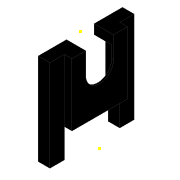
# Autodesk Inventor part: vertical_face_block
Saved by Autodesk Inventor 2019 (Build 230136000, 136)
## iProperties
Created: 2023-11-20
Part Number: vertical_face_block
Material: Aluminum 6061
Document SubType Name: Modeling
Designer: prich
Density: 2.7 g/cm^3
Appearance: Aluminum - Flat
Mass: 329.506 g
Surface Area: 342.022 cm^2
Volume: 122.039 cm^3
Author: prich
Autodesk Inventor part; units mm, degrees
ref_plane "YZ Plane" through (0, 0, 0) normal (1, 0, 0) x (0, 1, 0)
ref_plane "XZ Plane" through (0, 0, 0) normal (0, 1, 0) x (-1, 0, 0)
ref_plane "XY Plane" through (0, 0, 0) normal (0, 0, 1) x (1, 0, 0)
sketch "Sketch1" plane through (0, 0, 0) normal (0, 1, 0) x (-1, 0, 0)
  line L0 (0.0752, 55.5625) -> (-25.3248, 55.5625)
  line L1 (-25.3248, 55.5625) -> (-25.3248, -55.5625)
  line L2 (-25.3248, -55.5625) -> (0.0752, -55.5625)
  line L3 (0.0752, -55.5625) -> (0.0752, 55.5625)
  line L4 (54.9786, 0) -> (-47.41, 0) construction
  point P0 (0, 0)
  dimension "d0" = 111.125
  dimension "d1" = 25.4
  constraints: 10 end point, 2 horizontal, 2 parallel, 1 perpendicular, 1 other
  measures "d0" distance between parallel lines of L2 L0
  measures "d1" distance between parallel lines of L1 L3
extrude "Extrusion1" add sketch "Sketch1" along normal blind 120.65
sketch "Sketch2" plane through (25.3248, 0, 55.5625) normal (1, 0, 0) x (0, 0, -1)
  line L0 (55.5625, 0) -> (55.5625, 120.65) construction
  line L1 (0, 120.65) -> (111.125, 120.65) construction
  line L2 (19.05, 120.65) -> (92.075, 120.65)
  line L3 (92.075, 120.65) -> (92.075, 38.1)
  line L4 (92.075, 38.1) -> (19.05, 38.1)
  line L5 (19.05, 38.1) -> (19.05, 120.65)
  line L6 (19.05, 38.1) -> (19.05, 0)
  line L7 (0, 0) -> (111.125, 0) projected
  line L8 (92.075, 38.1) -> (92.075, 0)
  dimension "d4" = 82.55
  dimension "d10" = 73.025
  constraints: 14 end point, 3 parallel, 3 point on line, 1 horizontal, 1 midpoint, 1 perpendicular, 1 vertical, 1 other
  measures "d4" distance between parallel lines of L4 L1
  measures "d10" distance between parallel lines of L3 L5
extrude "Extrusion2" cut sketch "Sketch2" against normal blind 120.65 contours L4 L8 L7 L6
sketch "Sketch3" plane through (25.3248, 0, -55.5625) normal (1, 0, 0) x (0, 0, -1)
  line L0 (-92.075, 38.1) -> (-92.075, 120.65) projected
  line L1 (-19.05, 120.65) -> (-19.05, 38.1) projected
  line L2 (0, 0) -> (0, 120.65) projected
  line L3 (-111.125, 120.65) -> (0, 120.65) construction
  line L4 (-111.125, 0) -> (0, 0) projected
  line L5 (-111.125, 0) -> (-111.125, 120.65) projected
  line L6 (-19.05, 38.1) -> (-19.05, 0) projected
  line L7 (-92.075, 120.65) -> (-19.05, 120.65)
  line L8 (-19.05, 120.65) -> (-19.05, 38.1)
  line L9 (-19.05, 38.1) -> (-92.075, 38.1)
  line L10 (-92.075, 38.1) -> (-92.075, 120.65)
  line L11 (-92.075, 0) -> (-92.075, 38.1) projected
  line L12 (-111.125, 120.65) -> (-92.075, 120.65)
  line L13 (-92.075, 120.65) -> (-92.075, 0)
  line L14 (-92.075, 0) -> (-111.125, 0)
  line L15 (-111.125, 0) -> (-111.125, 120.65)
  line L16 (-19.05, 120.65) -> (0, 120.65)
  line L17 (0, 120.65) -> (0, 0)
  line L18 (0, 0) -> (-19.05, 0)
  line L19 (-19.05, 0) -> (-19.05, 120.65)
  point P0 (-55.5625, 0)
  constraints: 24 end point, 6 parallel, 3 horizontal, 3 perpendicular
extrude "Extrusion3" cut sketch "Sketch3" against normal blind 10 contours L11 L4 L5 L12 L0 | L1 L16 L2 L4 L6
sketch "Sketch4" plane through (-0.0752, 0, 55.5625) normal (-1, 0, 0) x (0, 0, 1)
  line L0 (-92.075, 0) -> (-92.075, 38.1) projected
  line L1 (-92.075, 38.1) -> (-19.05, 38.1) projected
  line L2 (-19.05, 38.1) -> (-19.05, 0) projected
  line L3 (-19.05, 0) -> (0, 0) projected
  line L4 (0, 0) -> (0, 120.65) projected
  line L5 (-111.125, 120.65) -> (0, 120.65) projected
  line L6 (-111.125, 0) -> (-111.125, 120.65) projected
  line L7 (-111.125, 0) -> (-92.075, 0) projected
  line L8 (-55.5625, 0) -> (-55.5625, 120.65) construction
  line L9 (-111.125, 120.65) -> (0, 120.65) construction
  line L10 (-88.9, 107.95) -> (-22.225, 107.95)
  line L11 (-22.225, 107.95) -> (-22.225, 50.8)
  line L12 (-22.225, 50.8) -> (-88.9, 50.8)
  line L13 (-88.9, 50.8) -> (-88.9, 107.95)
  dimension "d9" = 66.675
  dimension "d11" = 12.7
  dimension "d12" = 12.7
  constraints: 10 end point, 2 parallel, 1 horizontal, 1 midpoint, 1 perpendicular, 1 other
  measures "d9" distance between parallel lines of L11 L13
  measures "d11" distance between parallel lines of L1 L12
  measures "d12" distance between parallel lines of L10 L5
extrude "Extrusion4" cut sketch "Sketch4" against normal blind 23 contours L10 L11 L12 L13
sketch "Sketch5" plane through (25.3248, 38.1, 36.5125) normal (1, 0, 0) x (0, 0, -1)
  line L0 (36.5125, -38.1) -> (36.5125, 82.55) construction
  line L1 (0, 82.55) -> (73.025, 82.55) construction
  line L2 (18.2562, 82.55) -> (54.7687, 82.55)
  line L3 (54.7687, 82.55) -> (54.7687, 53.975)
  line L4 (54.7687, 53.975) -> (18.2562, 53.975)
  line L5 (18.2562, 53.975) -> (18.2562, 82.55)
  circle A0 centre (36.5125, 53.975) radius 18.2563
  dimension "d16" = 36.5125
  dimension "d17" = 28.575
  constraints: 10 end point, 2 midpoint, 2 parallel, 1 horizontal, 1 horizontal alignment, 1 perpendicular, 1 point on line, 3 other
  measures "d16" distance between parallel lines of L3 L5
  measures "d17" distance between parallel lines of L4 L1
fillet "Fillet1" radius 3.175 4 edges at (11.4248, 107.95, 33.3375) (11.4248, 50.8, 33.3375) (11.4248, 50.8, -33.3375) (11.4248, 107.95, -33.3375)
extrude "Extrusion5" cut sketch "Sketch5" against normal blind 25.4
sketch "Sketch6" plane through (25.3248, 38.1, 36.5125) normal (1, 0, 0) x (0, 0, -1)
  point P0 (36.5125, -38.1)
sketch "Sketch7" plane through (0, 120.65, 0) normal (0, 1, 0) x (1, 0, 0)
  point P0 (0, 0)
  point P1 (6.7165, -47.6926)
body "Solid1"
